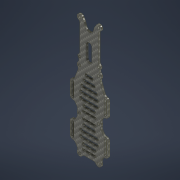
# Autodesk Inventor part: 10inchtopplatetenten
Saved by Autodesk Inventor 2021 (Build 250183000, 183)
## iProperties
Created: 2020-05-02
Part Number: 10inchtopplatetenten
Material: Generic
Document SubType Name: Modeling
Designer: Logan
Density: 1 g/cm^3
Appearance: Carbon Fiber 1
Mass: 10.2969 g
Surface Area: 101.618 cm^2
Volume: 10.2969 cm^3
Author: Logan
Autodesk Inventor part; units mm, degrees
ref_plane "YZ Plane" through (0, 0, 0) normal (1, 0, 0) x (0, 1, 0)
ref_plane "XZ Plane" through (0, 0, 0) normal (0, 1, 0) x (-1, 0, 0)
ref_plane "XY Plane" through (0, 0, 0) normal (0, 0, 1) x (1, 0, 0)
sketch "Sketch1" plane through (0, 0, 0) normal (0, 0, 1) x (1, 0, 0)
  line L0 (-13.5, -30) -> (13.5, -30) construction
  line L1 (13.5, -30) -> (13.5, 30)
  line L2 (13.5, 30) -> (-13.5, 30) construction
  line L3 (-13.5, 30) -> (-13.5, -30)
  line L4 (-13.5, -30) -> (13.5, 30) construction
  line L5 (13.5, -30) -> (-13.5, 30) construction
  line L6 (-13.5, -30) -> (13.5, -30) construction
  line L7 (13.5, -30) -> (13.5, -80) construction
  line L8 (13.5, -80) -> (-13.5, -80) construction
  line L9 (-13.5, -80) -> (-13.5, -30) construction
  line L10 (-13.5, 30) -> (13.5, 30)
  line L11 (13.5, 30) -> (13.5, 90) construction
  line L12 (13.5, 90) -> (-13.5, 90) construction
  line L13 (-13.5, 90) -> (-13.5, 30) construction
  circle A0 centre (-13.5, 90) radius 1.5
  circle A1 centre (13.5, 90) radius 1.5
  circle A2 centre (-13.5, 30) radius 1.5
  circle A3 centre (13.5, 30) radius 1.5
  circle A4 centre (13.5, -30) radius 1.5
  circle A5 centre (-13.5, -30) radius 1.5
  circle A6 centre (-13.5, -80) radius 1.5
  circle A7 centre (13.5, -80) radius 1.5
  line L14 (-13.5, 90) -> (-13.5, 30) construction
  line L15 (13.5, 30) -> (13.5, 90) construction
  line L16 (13.5, 30) -> (73.5, 30) construction
  line L17 (-13.5, 30) -> (13.5, 90) construction
  line L18 (-13.5, 90) -> (13.5, 30) construction
  line L19 (-13.5, 30) -> (13.5, 30) construction
  line L20 (-13.5, 30) -> (-13.5, -80) construction
  line L21 (0, 0) -> (0, 8.9459)
  line L22 (-13.5, 90) -> (13.5, 90)
  line L23 (13.5, 90) -> (13.5, 30)
  line L24 (13.5, 30) -> (-13.5, 30)
  line L25 (-13.5, 30) -> (-13.5, 90)
  circle A8 centre (-13.5, 90) radius 4
  circle A9 centre (13.5, 90) radius 4
  line L26 (0, 90) -> (0, 78)
  line L27 (-9.5, 90) -> (-5.7182, 88.5) construction
  line L28 (-5.7182, 88.5) -> (-8.1516, 78.1147) construction
  line L29 (-8.1516, 78.1147) -> (0, 78) construction
  spline S0 degree 3 poles (-9.5, 90) (-5.7182, 88.5) (-8.1516, 78.1147) (0, 78) knots 1 1 1 1 2 2 2 2
  line L30 (9.5, 90) -> (5.7182, 88.5) construction
  line L31 (5.7182, 88.5) -> (8.1516, 78.1147) construction
  line L32 (8.1516, 78.1147) -> (0, 78) construction
  spline S1 degree 3 poles (9.5, 90) (5.7182, 88.5) (8.1516, 78.1147) (0, 78) knots 1 1 1 1 2 2 2 2
  line L33 (0, 60) -> (0, 52)
  line L34 (0, 61) -> (0, 43) construction
  line L35 (-4, 61) -> (-4, 43)
  line L36 (4, 43) -> (4, 61)
  arc A10 (4, 61) -> (-4, 61) centre (0, 61) ccw
  arc A11 (-4, 43) -> (4, 43) centre (0, 43) ccw
  line L37 (-13.5, -30) -> (13.5, -30)
  line L38 (13.5, -30) -> (13.5, -80)
  line L39 (13.5, -80) -> (-13.5, -80)
  line L40 (-13.5, -80) -> (-13.5, -30)
  circle A12 centre (-13.5, 30) radius 4
  circle A13 centre (13.5, 30) radius 4
  circle A14 centre (-13.5, -30) radius 4
  circle A15 centre (13.5, -30) radius 4
  circle A16 centre (13.5, -80) radius 4
  circle A17 centre (-13.5, -80) radius 4
  line L41 (13.5, -55) -> (23.5, -55)
  line L42 (13.5, -30) -> (13.5, -5)
  line L43 (13.5, -5) -> (23.5, -5)
  line L44 (23.5, 4) -> (23.5, -14) construction
  line L45 (22, 4) -> (22, -14)
  line L46 (25, -14) -> (25, 4)
  arc A18 (25, 4) -> (22, 4) centre (23.5, 4) ccw
  arc A19 (22, -14) -> (25, -14) centre (23.5, -14) ccw
  line L47 (23.5, -5) -> (41.5, -5) construction
  line L48 (23.5, -46) -> (23.5, -64) construction
  line L49 (22, -46) -> (22, -64)
  line L50 (25, -64) -> (25, -46)
  arc A20 (25, -46) -> (22, -46) centre (23.5, -46) ccw
  arc A21 (22, -64) -> (25, -64) centre (23.5, -64) ccw
  line L51 (23.5, -55) -> (41.5, -55) construction
  line L52 (23.5, -14) -> (23.5, 4) construction
  line L53 (27.5, -14) -> (27.5, 4)
  line L54 (19.5, 4) -> (19.5, -14)
  arc A22 (19.5, -14) -> (27.5, -14) centre (23.5, -14) ccw
  arc A23 (27.5, 4) -> (19.5, 4) centre (23.5, 4) ccw
  line L55 (23.5, -64) -> (23.5, -46) construction
  line L56 (27.5, -64) -> (27.5, -46)
  line L57 (19.5, -46) -> (19.5, -64)
  arc A24 (19.5, -64) -> (27.5, -64) centre (23.5, -64) ccw
  arc A25 (27.5, -46) -> (19.5, -46) centre (23.5, -46) ccw
  line L58 (-22, 4) -> (-22, -14)
  line L59 (-25, -14) -> (-25, 4)
  arc A26 (-22, 4) -> (-25, 4) centre (-23.5, 4) ccw
  arc A27 (-25, -14) -> (-22, -14) centre (-23.5, -14) ccw
  line L60 (-22, -46) -> (-22, -64)
  line L61 (-25, -64) -> (-25, -46)
  arc A28 (-22, -46) -> (-25, -46) centre (-23.5, -46) ccw
  arc A29 (-25, -64) -> (-22, -64) centre (-23.5, -64) ccw
  line L62 (-27.5, -14) -> (-27.5, 4)
  arc A30 (-27.5, -14) -> (-19.5, -14) centre (-23.5, -14) ccw
  arc A31 (-19.5, 4) -> (-27.5, 4) centre (-23.5, 4) ccw
  line L63 (-27.5, -64) -> (-27.5, -46)
  line L64 (-19.5, -46) -> (-19.5, -64)
  arc A32 (-27.5, -64) -> (-19.5, -64) centre (-23.5, -64) ccw
  arc A33 (-19.5, -46) -> (-27.5, -46) centre (-23.5, -46) ccw
  line L65 (-19.5, -14) -> (-19.5, 4)
  line L66 (-23.5, -64) -> (-13.5, -80)
  line L67 (13.5, -80) -> (23.5, -64)
  line L68 (23.5, -46) -> (13.5, -30)
  line L69 (13.5, -30) -> (23.5, -14)
  line L70 (23.5, 4) -> (13.5, 30)
  line L71 (-13.5, 30) -> (-23.5, 4)
  line L72 (-23.5, -46) -> (-13.5, -30)
  line L73 (-23.5, -14) -> (-13.5, -30)
  line L74 (-23.5, -46) -> (-23.5, -64)
  line L75 (-23.5, 4) -> (-23.5, -14)
  line L76 (23.5, 4) -> (23.5, -14)
  line L77 (23.5, -46) -> (23.5, -64)
  line L78 (-5.02, -74.7) -> (-13.5, -61.132)
  line L79 (-13.5, -61.132) -> (-13.5, -48.868)
  line L80 (-13.5, -48.868) -> (-1.7075, -30)
  line L81 (-1.7075, -30) -> (-13.5, -11.132)
  line L82 (-13.5, -11.132) -> (-13.5, 2.1432)
  line L83 (-13.5, 2.1432) -> (-4.1665, 26.4102)
  line L84 (5.02, -24.7) -> (13.5, -11.132)
  line L85 (13.5, -11.132) -> (13.5, 2.1432)
  line L86 (13.5, 2.1432) -> (4.1665, 26.4102)
  line L87 (5.02, -35.3) -> (13.5, -48.868)
  line L88 (13.5, -48.868) -> (13.5, -61.132)
  line L89 (13.5, -61.132) -> (5.02, -74.7)
  line L90 (5.02, -24.7) -> (1.7075, -30)
  line L91 (5.02, -35.3) -> (1.7075, -30)
  line L92 (-13.5, -80) -> (-13.5, -68)
  line L93 (-13.5, -68) -> (13.5, -68)
  line L94 (-13.5, 30) -> (-13.5, 24)
  line L95 (-13.5, 24) -> (13.5, 24)
  line L96 (0, -30) -> (0, -38)
  line L97 (0, -38) -> (0, -46)
  line L98 (0, -46) -> (0, -54)
  line L99 (0, -54) -> (0, -62)
  line L100 (0, -62) -> (0, -73.25)
  line L101 (0, -30) -> (0, -22)
  line L102 (0, -22) -> (0, -14)
  line L103 (0, -14) -> (0, -6)
  line L104 (0, -6) -> (0, 2)
  line L105 (0, 2) -> (0, 10)
  line L106 (0, 10) -> (0, 18)
  line L107 (-11, -36) -> (11, -36)
  line L108 (11, -36) -> (11, -40)
  line L109 (11, -40) -> (-11, -40)
  line L110 (-11, -40) -> (-11, -36)
  line L111 (-11, -36) -> (11, -40) construction
  line L112 (11, -36) -> (-11, -40) construction
  line L113 (-17.5, -44) -> (17.5, -44)
  line L114 (17.5, -44) -> (17.5, -48)
  line L115 (17.5, -48) -> (-17.5, -48)
  line L116 (-17.5, -48) -> (-17.5, -44)
  line L117 (-17.5, -44) -> (17.5, -48) construction
  line L118 (17.5, -44) -> (-17.5, -48) construction
  line L119 (-17.5, -56) -> (17.5, -56)
  line L120 (17.5, -56) -> (17.5, -52)
  line L121 (17.5, -52) -> (-17.5, -52)
  line L122 (-17.5, -52) -> (-17.5, -56)
  line L123 (-17.5, -56) -> (17.5, -52) construction
  line L124 (17.5, -56) -> (-17.5, -52) construction
  line L125 (-17.5, -60) -> (17.5, -60)
  line L126 (17.5, -60) -> (17.5, -64)
  line L127 (17.5, -64) -> (-17.5, -64)
  line L128 (-17.5, -64) -> (-17.5, -60)
  line L129 (-17.5, -60) -> (17.5, -64) construction
  line L130 (17.5, -60) -> (-17.5, -64) construction
  line L131 (-12, -24) -> (12, -24)
  line L132 (12, -24) -> (12, -20)
  line L133 (12, -20) -> (-12, -20)
  line L134 (-12, -20) -> (-12, -24)
  line L135 (-12, -24) -> (12, -20) construction
  line L136 (12, -24) -> (-12, -20) construction
  line L137 (-16, -16) -> (16, -16)
  line L138 (16, -16) -> (16, -12)
  line L139 (16, -12) -> (-16, -12)
  line L140 (-16, -12) -> (-16, -16)
  line L141 (-16, -16) -> (16, -12) construction
  line L142 (16, -16) -> (-16, -12) construction
  line L143 (-17.5, -8) -> (17.5, -8)
  line L144 (17.5, -8) -> (17.5, -4)
  line L145 (17.5, -4) -> (-17.5, -4)
  line L146 (-17.5, -4) -> (-17.5, -8)
  line L147 (-17.5, -8) -> (17.5, -4) construction
  line L148 (17.5, -8) -> (-17.5, -4) construction
  line L149 (-16, 0) -> (16, 0)
  line L150 (16, 0) -> (16, 4)
  line L151 (16, 4) -> (-16, 4)
  line L152 (-16, 4) -> (-16, 0)
  line L153 (-16, 0) -> (16, 4) construction
  line L154 (16, 0) -> (-16, 4) construction
  line L155 (-14, 8) -> (14, 8)
  line L156 (14, 8) -> (14, 12)
  line L157 (14, 12) -> (-14, 12)
  line L158 (-14, 12) -> (-14, 8)
  line L159 (-14, 8) -> (14, 12) construction
  line L160 (14, 8) -> (-14, 12) construction
  line L161 (-12, 16) -> (12, 16)
  line L162 (12, 16) -> (12, 20)
  line L163 (12, 20) -> (-12, 20)
  line L164 (-12, 20) -> (-12, 16)
  line L165 (-12, 16) -> (12, 20) construction
  line L166 (12, 16) -> (-12, 20) construction
  line L167 (0, -30) -> (0, -34.75)
  line L168 (0, -30) -> (0, -25.25)
  line L169 (9, -34.75) -> (-9, -34.75) construction
  line L170 (9, -33.5) -> (-9, -33.5)
  line L171 (-9, -36) -> (9, -36)
  arc A34 (9, -36) -> (9, -33.5) centre (9, -34.75) ccw
  arc A35 (-9, -33.5) -> (-9, -36) centre (-9, -34.75) ccw
  line L172 (9, -25.25) -> (-9, -25.25) construction
  line L173 (9, -24) -> (-9, -24)
  line L174 (-9, -26.5) -> (9, -26.5)
  arc A36 (9, -26.5) -> (9, -24) centre (9, -25.25) ccw
  arc A37 (-9, -24) -> (-9, -26.5) centre (-9, -25.25) ccw
  line L175 (9, -73.25) -> (-9, -73.25) construction
  line L176 (9, -72) -> (-9, -72)
  line L177 (-9, -74.5) -> (9, -74.5)
  arc A38 (9, -74.5) -> (9, -72) centre (9, -73.25) ccw
  arc A39 (-9, -72) -> (-9, -74.5) centre (-9, -73.25) ccw
  line L178 (-13.5, 90) -> (-13.5, 41)
  line L179 (-13.5, 41) -> (13.5, 41)
  circle A40 centre (-13.5, 41) radius 1.5
  circle A41 centre (-13.5, 41) radius 3
  circle A42 centre (13.5, 41) radius 1.5
  circle A43 centre (13.5, 41) radius 3
  point P0 (-13.5, 60)
  point P1 (13.5, 60)
  point P2 (0, 60)
  point P3 (-13.5, -25)
  point P4 (-13.5, 86)
  point P5 (13.5, 86)
  point P6 (9.5, 90)
  point P7 (9.5, 90)
  point P8 (-9.5, 90)
  point P9 (-9.5, 90)
  point P10 (9.5, 90)
  point P11 (-13.5, -34)
  point P12 (-13.5, -38)
  point P13 (-13.5, -56)
  point P14 (-13.5, -76)
  point P15 (-9.5, -80)
  point P16 (9.5, -80)
  point P17 (13.5, -76)
  point P18 (13.5, -56)
  point P19 (13.5, -38)
  point P20 (13.5, -34)
  point P21 (13.5, -26)
  point P22 (13.5, -13.5)
  point P23 (13.5, 4.5)
  point P24 (13.5, 26)
  point P25 (13.5, 34)
  point P26 (13.5, 31.5)
  point P27 (12, 30)
  point P28 (-12, 30)
  point P29 (-13.5, 31.5)
  point P30 (-13.5, 34)
  point P31 (-13.5, 26)
  point P32 (-13.5, 4.5)
  point P33 (-13.5, -13.5)
  point P34 (-13.5, -26)
  point P35 (13.5, 28.5)
  point P36 (-13.5, 28.5)
  point P37 (15.62, -76.608)
  point P38 (21.38, -67.392)
  point P39 (21.38, -42.608)
  point P40 (15.62, -33.392)
  point P41 (15.62, -26.608)
  point P42 (21.38, -17.392)
  point P43 (22.0641, 7.7334)
  point P44 (14.9359, 26.2666)
  point P45 (13.5, -28.5)
  point P46 (13.5, -31.5)
  point P47 (-21.38, -17.392)
  point P48 (-15.62, -26.608)
  point P49 (-15.62, -33.392)
  point P50 (-21.38, -42.608)
  point P51 (-21.38, -67.392)
  point P52 (-15.62, -76.608)
  point P53 (-13.5, -31.5)
  point P54 (-13.5, -28.5)
  point P55 (-14.9359, 26.2666)
  point P56 (-22.0641, 7.7334)
  point P57 (13.5, -52)
  point P58 (-13.5, -52)
  point P59 (-12.9575, -48)
  point P60 (12.9575, -48)
  point P61 (-5.4575, -24)
  point P62 (5.4575, -24)
  point P63 (-12.9575, -12)
  point P64 (-13.5, -8)
  point P65 (13.5, -8)
  point P66 (12.9575, -12)
  point P67 (6.632, 20)
  point P68 (-6.632, 20)
  point P69 (-5.0935, 24)
  point P70 (5.0935, 24)
  point P71 (12.7859, 4)
  point P72 (-12.7859, 4)
  point P73 (-11.2474, 8)
  point P74 (11.2474, 8)
  point P75 (-9.7089, 12)
  point P76 (-8.1705, 16)
  point P77 (8.1705, 16)
  point P78 (9.7089, 12)
  point P79 (13.5, -4)
  point P80 (-13.5, -4)
  point P81 (-13.5, 0)
  point P82 (13.5, 0)
  point P83 (-10.4575, -16)
  point P84 (10.4575, -16)
  point P85 (7.9575, -20)
  point P86 (-7.9575, -20)
  point P87 (-11.7075, -64)
  point P88 (11.7075, -64)
  point P89 (9.2075, -68)
  point P90 (-9.2075, -68)
  point P91 (7.9575, -40)
  point P92 (10.4575, -44)
  point P93 (-10.4575, -44)
  point P94 (-7.9575, -40)
  point P95 (5.4575, -36)
  point P96 (-5.4575, -36)
  point P97 (13.5, -56)
  point P98 (13.5, -60)
  point P99 (-13.5, -60)
  point P100 (-13.5, -56)
  point P101 (-13.5, 44)
  point P102 (-13.5, 38)
  point P103 (13.5, 38)
  point P104 (13.5, 44)
  dimension "d40" = 8
  dimension "d0" = 27
  dimension "d1" = 60
  dimension "d2" = 27
  dimension "d3" = 50
  dimension "d4" = 27
  dimension "d5" = 60
  dimension "d6" = 3
  dimension "d7" = 3
  dimension "d8" = 3
  dimension "d9" = 3
  dimension "d10" = 3
  dimension "d11" = 3
  dimension "d12" = 3
  dimension "d13" = 3
  dimension "d17" = 60
  dimension "d18" = 90
  dimension "d41" = 8
  dimension "d42" = 12
  dimension "d43" = 8
  dimension "d44" = 9
  dimension "d45" = 8
  dimension "d46" = 8
  dimension "d47" = 8
  dimension "d48" = 8
  dimension "d49" = 8
  dimension "d50" = 8
  dimension "d51" = 8
  dimension "d52" = 10
  dimension "d53" = 25
  dimension "d54" = 10
  dimension "d55" = 9
  dimension "d56" = 90
  dimension "d57" = 3
  dimension "d58" = 9
  dimension "d59" = 90
  dimension "d60" = 3
  dimension "d61" = 8
  dimension "d62" = 8
  dimension "d65" = 10
  dimension "d66" = 10
  dimension "d67" = 10
  dimension "d70" = 12
  dimension "d71" = 6
  dimension "d72" = 8
  dimension "d73" = 8
  dimension "d74" = 8
  dimension "d75" = 8
  dimension "d76" = 11.25
  dimension "d77" = 8
  dimension "d78" = 8
  dimension "d79" = 8
  dimension "d80" = 8
  dimension "d81" = 8
  dimension "d82" = 8
  dimension "d85" = 22
  dimension "d86" = 4
  dimension "d87" = 35
  dimension "d88" = 4
  dimension "d89" = 35
  dimension "d90" = 4
  dimension "d91" = 35
  dimension "d92" = 4
  dimension "d95" = 24
  dimension "d96" = 4
  constraints: 376 end point, 48 point on circle, 43 centre point, 40 parallel, 38 midpoint, 32 tangent, 27 perpendicular, 26 symmetric about line, 23 point on line, 20 coincident, 20 horizontal, 9 vertical, 3 collinear, 26 other
  measures "d0" distance of L2.end L1.end
  measures "d1" distance of L1.end L0.end
  measures "d2" distance of L7.end L8.end
  measures "d3" distance of L6.end L7.end
  measures "d4" distance of L12.end L11.end
  measures "d5" distance of L11.end L10.end
  measures "d6" diameter of A0
  measures "d7" diameter of A1
  measures "d8" diameter of A2
  measures "d9" diameter of A3
  measures "d10" diameter of A4
  measures "d11" diameter of A5
  measures "d12" diameter of A6
  measures "d13" diameter of A7
  measures "d17" distance of L15.start L15.end
  measures "d18" angle of L16 L15
  measures "d41" diameter of A9
  measures "d42" distance of L26.start L26.end
  measures "d43" distance of L33.start L33.end
  measures "d44" distance of L33.end L34.end
  measures "d45" diameter of A11
  measures "d46" diameter of A12
  measures "d47" diameter of A13
  measures "d48" diameter of A14
  measures "d49" diameter of A15
  measures "d50" diameter of A16
  measures "d51" diameter of A17
  measures "d52" distance of L41.start L41.end
  measures "d53" distance of L42.start L42.end
  measures "d54" distance of L42.end L43.end
  measures "d55" distance of L43.end L44.end
  measures "d56" angle of L44 L47
  measures "d57" diameter of A19
  measures "d58" distance of L41.end L48.end
  measures "d59" angle of L48 L51
  measures "d60" diameter of A21
  measures "d61" diameter of A23
  measures "d62" diameter of A25
  measures "d65" distance between parallel lines of L66 L78
  measures "d66" distance between parallel lines of L69 L84
  measures "d67" distance between parallel lines of L68 L87
  measures "d70" distance of L66.end L92.end
  measures "d71" distance of L71.start L94.end
  measures "d72" distance of L96.start L96.end
  measures "d73" distance of L96.end L97.end
  measures "d74" distance of L97.end L98.end
  measures "d75" distance of L98.end L99.end
  measures "d76" distance of L99.end L100.end
  measures "d77" distance of L96.start L101.end
  measures "d78" distance of L101.end L102.end
  measures "d79" distance of L102.end L103.end
  measures "d80" distance of L103.end L104.end
  measures "d81" distance of L104.end L105.end
  measures "d82" distance of L105.end L106.end
  measures "d85" distance of L108.end L109.end
  measures "d86" distance of L107.end L108.end
  measures "d87" distance of L114.end L115.end
  measures "d88" distance of L113.end L114.end
  measures "d89" distance of L121.end L120.end
  measures "d90" distance of L120.end L119.end
  measures "d91" distance of L126.end L127.end
  measures "d92" distance of L125.end L126.end
  measures "d95" distance of L133.end L132.end
  measures "d96" distance of L132.end L131.end
extrude "Extrusion1" add sketch "Sketch1" along normal blind 2.5 contours A4 L37 A15 L1 | L1 A15 L69 A4 | A4 L38 A15 L37 | A4 L68 A15 L38 | A4 L69 A15 L68 | A15 L37 L90 L174 A36 L131 L132 L133 L84 L137 L1 | L1 L137 L138 L139 L143 L144 L43 L54 A22 L69 A15 | A15 L38 L113 L87 L109 L108 L107 A34 L170 L91 L37 | A15 L68 A25 L57 L41 L120 L121 L38 L115 L114 L113 | L137 L84 L139 L1 | L1 L139 L138 L137 | L91 L170 L96 L37 | L37 L101 L174 L90 | L113 L114 L115 L38 | L38 L115 L87 L113 | L68 A20 L49 L41 L57 A25 | A25 L56 A24 L67 A21 L50 A20 L68 | L69 A19 L46 A18 L70 A23 L53 A22 | A22 L54 L43 L45 A19 L69 | L139 L84 L1 | L137 L102 L103 L139 L84 | L96 L170 L80 L37 | L37 L81 L174 L101 | L38 L87 L115 | L87 L115 L98 L97 L113 | L133 L132 L131 L84 | L84 L131 L101 L102 L133 | L137 L81 L139 L103 L102 | L80 L170 A35 L107 L110 L109 L113 L40 A14 L37 | L37 A14 L3 L137 L81 L133 L134 L131 A37 L174 | L109 L97 L96 L107 L87 | L87 L107 L108 L109 | L97 L98 L115 L80 L113 | L57 A24 L67 A16 L38 L127 L126 L125 L119 L120 L41 | L41 L49 A21 L67 A24 L57 | L54 A23 L70 A18 L45 L43 | L43 L144 L145 L1 L149 L150 L151 L155 L156 L157 A13 L70 A23 L54 | L143 L103 L104 L145 L1 | L1 L43 L144 L143 | L102 L101 L131 L81 L133 | L137 L3 L139 L81 | A14 L40 A5 L37 | L37 A5 L3 A14 | L121 L120 L41 L38 | L38 L119 L99 L98 L121 | L109 L80 L107 L96 L97 | L80 L115 L40 L113 | L120 L119 L38 L41 | L43 L1 L145 L144 | L143 L3 L145 L104 L103 | L139 L3 L81 | L81 L131 L134 L133 | L137 L140 L139 L3 | L3 A14 L73 A30 L65 A31 L71 A12 L157 L158 L155 L151 L152 L149 L145 L146 L143 L139 L140 L137 | L3 A5 L73 A14 | A14 L72 A5 L40 | L40 L113 L116 L115 L121 L122 L119 L125 L128 L127 A17 L66 A32 L64 A33 L72 A14 | L80 L109 L110 L107 | L98 L99 L119 L40 L121 | L80 L40 L115 | L40 L115 L116 L113 | L67 A7 L38 A16 | A16 L39 A7 L67 | L70 A3 L23 A13 | A13 L1 A3 L70 | L143 L146 L145 L3 | L73 A5 L72 A14 | L40 L119 L122 L121 | A16 L39 A17 L40 L93 L78 L176 A39 L177 A38 L89 L38 | L38 A7 L39 A16 | A13 L10 A3 L1 | L1 L95 L3 A12 L10 A13 | L149 L21 L151 L86 L1 | L1 L151 L150 L149 | L73 A27 L58 A26 L71 A31 L65 A30 | A30 L62 A31 L71 A26 L59 A27 L73 | L72 A28 L61 A29 L66 A32 L63 A33 | A33 L64 A32 L66 A29 L60 A28 L72 | L125 L126 L127 L38 | L38 L89 L127 L100 L99 L125 | L93 L89 L127 L38 | L1 L157 L86 L161 L162 L163 L95 | A13 L23 A3 L10 | L10 A12 L25 A41 L179 A11 A43 L23 A13 | L86 L151 L1 | L149 L3 L83 L151 L21 | L149 L152 L151 L3 | L38 L127 L89 | L99 L100 L127 L78 L40 L125 | L40 L127 L128 L125 | A17 L66 A6 L39 | L39 A6 L40 A17 | L89 L176 L100 L93 | L157 L156 L155 L1 | L1 L155 L86 L157 | A12 L3 A2 L10 | L10 A2 L25 A12 | A43 L179 A42 L23 | L23 A42 A43 | L151 L86 L155 L1 | L3 L151 L83 | L78 L127 L40 | L40 A6 L66 A17 | L100 L176 L78 L93 | L86 L155 L21 L105 L106 L157 | L163 L162 L161 L86 | L86 L161 L83 L163 | L83 L163 L164 L161 L157 L3 L95 | L25 A2 L71 A12 | A12 L71 A2 L3 | A43 L23 A42 L179 | L179 A11 L36 A10 L35 A41 L25 A8 S0 S1 A9 L23 A43 | L3 L155 L83 L151 | L127 L78 L93 L40 | L106 L105 L21 L155 L83 L157 | L83 L161 L164 L163 | A41 L25 A40 | L25 A40 L179 A41 | L155 L158 L157 L3 | L3 L157 L83 L155 | A41 L179 A40 L25 | A9 L22 A1 L23 | L23 A1 L22 A9 | A8 L22 A0 L25 | L25 A0 L22 A8
fillet "Fillet4" radius 4 28 edges at (-21.38, -42.608, 1.25) (-15.62, -33.392, 1.25) (-15.62, -26.608, 1.25) (-21.38, -17.392, 1.25) (-22.0641, 7.7334, 1.25) (-14.9359, 26.2666, 1.25) (14.9359, 26.2666, 1.25) (22.0641, 7.7334, 1.25) (21.38, -17.392, 1.25) (15.62, -26.608, 1.25) (15.62, -33.392, 1.25) (21.38, -42.608, 1.25) (21.38, -67.392, 1.25) (15.62, -76.608, 1.25) (-15.62, -76.608, 1.25) (-21.38, -67.392, 1.25) (13.5, 34, 1.25) (-13.5, 86, 1.25) (-9.5, 90, 1.25) (9.5, 90, 1.25) (13.5, 86, 1.25) (9.5, -80, 1.25) (-9.5, -80, 1.25) (-13.5, 38, 1.25) (-13.5, 44, 1.25) (13.5, 38, 1.25) (13.5, 44, 1.25) (-13.5, 34, 1.25)
fillet "Fillet5" radius 1.6 44 edges at (-5.0935, 24, 1.25) (-6.632, 20, 1.25) (5.0935, 24, 1.25) (6.632, 20, 1.25) (-8.1705, 16, 1.25) (-9.7089, 12, 1.25) (-11.2474, 8, 1.25) (-12.7859, 4, 1.25) (-13.5, 0, 1.25) (-13.5, -4, 1.25) (-13.5, -8, 1.25) (-12.9575, -12, 1.25) (-13.5, -11.132, 1.25) (-10.4575, -16, 1.25) (-7.9575, -20, 1.25) (-7.9575, -40, 1.25) (-10.4575, -44, 1.25) (-12.9575, -48, 1.25) (-13.5, -48.868, 1.25) (-13.5, -52, 1.25) (-13.5, -56, 1.25) (-13.5, -60, 1.25) (-11.7075, -64, 1.25) (-9.2075, -68, 1.25) (11.7075, -64, 1.25) (13.5, -60, 1.25) (13.5, -56, 1.25) (13.5, -52, 1.25) (13.5, -48.868, 1.25) (10.4575, -44, 1.25) (7.9575, -40, 1.25) (7.9575, -20, 1.25) (10.4575, -16, 1.25) (13.5, -11.132, 1.25) (12.9575, -12, 1.25) (13.5, -8, 1.25) (13.5, -4, 1.25) (13.5, 0, 1.25) (12.7859, 4, 1.25) (11.2474, 8, 1.25) (9.7089, 12, 1.25) (8.1705, 16, 1.25) (9.2075, -68, 1.25) (12.9575, -48, 1.25)
body "Solid1"
